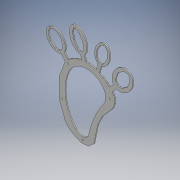
# Autodesk Inventor part: pata-carli
Saved by Autodesk Inventor 2018 (Build 220112000, 112)
## iProperties
Created: 2019-01-30
Part Number: pata-carli
Material: Generic
Document SubType Name: Modeling
Designer: Estudiante
Density: 1 g/cm^3
Appearance: Default
Author: Estudiante
Autodesk Inventor part; units mm, degrees
ref_plane "YZ Plane" through (0, 0, 0) normal (1, 0, 0) x (0, 1, 0)
ref_plane "XZ Plane" through (0, 0, 0) normal (0, 1, 0) x (-1, 0, 0)
ref_plane "XY Plane" through (0, 0, 0) normal (0, 0, 1) x (1, 0, 0)
sketch "Sketch1" plane through (0, 0, 0) normal (0, 1, 0) x (-1, 0, 0)
  line L0 (29.0554, 72.9814) -> (31.569, 71.953)
  line L1 (26.8219, 78.0587) -> (27.3884, 75.1254)
  line L2 (-19.8596, 89.1891) -> (-16.4882, 83.2487)
  line L3 (-14.1887, 81.7828) -> (-16.4882, 83.2487)
  line L4 (-11.9312, 81.6749) -> (-14.1887, 81.7828)
  line L5 (-10.0593, 82.9415) -> (-8.8581, 85.3896)
  line L6 (-11.9312, 81.6749) -> (-10.0593, 82.9415)
  line L7 (-8.8581, 85.3896) -> (-9.069, 92.2167)
  line L8 (-41.4432, 74.6738) -> (-35.9743, 70.6026)
  line L9 (-33.1014, 70.2673) -> (-35.9743, 70.6026)
  line L10 (-29.1988, 73.2448) -> (-28.7633, 76.1043)
  line L11 (-30.7221, 71.1952) -> (-33.1014, 70.2673)
  line L12 (-30.7221, 71.1952) -> (-29.1988, 73.2448)
  line L13 (-7.492, 12.8385) -> (-5.9259, 5.1471)
  line L14 (-9.7228, 24.2495) -> (-7.492, 12.8385)
  line L15 (-14.8718, 34.6743) -> (-9.7228, 24.2495)
  arc A0 (0, 8.9928) -> (-17.0107, 47.8982) centre (-95.643, -9.6539) ccw
  line L16 (-22.5775, 43.3812) -> (-14.8718, 34.6743)
  line L17 (31.569, 71.953) -> (34.5464, 72.1968)
  line L18 (29.1542, 84.4544) -> (26.8219, 78.0587)
  line L19 (34.5464, 72.1968) -> (40.0784, 76.1644)
  ellipse E0 centre (34.1936, 79.8506) end of major axis (26.5803, 71.3598) minor radius 9.1242 (28.5488, 70.094) -> (25.1982, 73.0271) ccw
  line L20 (40.0784, 76.1644) -> (42.4108, 82.5601)
  line L21 (34.6862, 88.422) -> (29.1542, 84.4544)
  line L22 (37.6637, 88.6658) -> (34.6862, 88.422)
  line L23 (42.4108, 82.5601) -> (41.8442, 85.4933)
  line L24 (38.9769, 87.7295) -> (37.6637, 88.6658)
  line L25 (41.8442, 85.4933) -> (40.5696, 86.5213)
  line L26 (9.0686, 82.2611) -> (11.3681, 83.5573)
  line L27 (4.8438, 86.2831) -> (5.5377, 83.7363)
  line L28 (12.3808, 100.1152) -> (10.0813, 98.819)
  line L29 (10.0813, 98.819) -> (6.1114, 93.1156)
  line L30 (13.4287, 100.083) -> (12.3808, 100.1152)
  line L31 (15.9117, 98.6399) -> (15.1525, 99.3628)
  line L32 (16.6056, 96.0931) -> (15.9117, 98.6399)
  line L33 (6.1114, 93.1156) -> (4.8438, 86.2831)
  ellipse E1 centre (10.6599, 91.6284) end of major axis (5.8794, 80.032) minor radius 8.4665 (8.3836, 79.5956) -> (4.3048, 81) ccw
  line L34 (15.3381, 89.2606) -> (16.6056, 96.0931)
  line L35 (11.3681, 83.5573) -> (15.3381, 89.2606)
  line L36 (6.6564, 75.1739) -> (11.5071, 73.874)
  line L37 (17.2873, 71.1447) -> (11.5071, 73.874)
  line L38 (21.4394, 68.1777) -> (17.2873, 71.1447)
  line L39 (21.4394, 68.1777) -> (17.2873, 71.1447)
  line L40 (25.1982, 73.0271) -> (21.4394, 68.1777)
  line L41 (29.0554, 72.9814) -> (27.3884, 75.1254)
  line L42 (28.5488, 70.094) -> (24.4313, 64.7818)
  line L43 (30.8467, 47.8624) -> (24.4313, 64.7818)
  line L44 (24.4313, 64.7818) -> (30.8467, 47.8624)
  line L45 (-43.9252, 81.0239) -> (-41.4432, 74.6738)
  line L46 (-28.7633, 76.1043) -> (-31.2452, 82.4543)
  ellipse E2 centre (-35.9971, 78.0469) end of major axis (-28.1232, 67.9201) minor radius 9.7067 (-26.561, 69.5776) -> (-29.6965, 66.9839) ccw
  line L47 (-43.4897, 83.8833) -> (-43.9252, 81.0239)
  line L48 (-31.2452, 82.4543) -> (-36.7141, 86.5255)
  line L49 (-42.5628, 85.1304) -> (-43.4897, 83.8833)
  line L50 (-36.7141, 86.5255) -> (-39.5871, 86.8608)
  line L51 (-39.5871, 86.8608) -> (-41.0347, 86.2963)
  ellipse E3 centre (-14.6571, 90.5791) end of major axis (-17.7823, 101.3962) minor radius 7.7041 (-10.1842, 80.3645) -> (-13.4664, 79.5698) ccw
  line L52 (-20.0705, 96.0162) -> (-19.8596, 89.1891)
  line L53 (-20.0705, 96.0162) -> (-19.8596, 89.1891)
  line L54 (-9.069, 92.2167) -> (-12.4404, 98.1571)
  line L55 (-12.4404, 98.1571) -> (-14.7399, 99.623)
  line L56 (-18.8693, 98.4643) -> (-20.0705, 96.0162)
  line L57 (-14.7399, 99.623) -> (-15.9985, 99.6831)
  line L58 (-17.8256, 99.1705) -> (-18.8693, 98.4643)
  line L59 (-26.561, 69.5776) -> (-22.2934, 65.085)
  line L60 (-19.5653, 67.6766) -> (-22.2934, 65.085)
  line L61 (-22.2934, 65.085) -> (-19.5653, 67.6766)
  line L62 (7.0212, 82.3239) -> (9.0686, 82.2611)
  line L63 (-1.0343, 75.4482) -> (2.443, 75.5931)
  arc A1 (20.9491, 56.7394) -> (-17.0336, 58.9292) centre (1.4249, 48.592) ccw
  line L64 (-1.0343, 75.4482) -> (-5.3277, 74.7251)
  line L65 (-5.3277, 74.7251) -> (-8.4472, 73.7874)
  line L66 (-10.1842, 80.3645) -> (-8.4472, 73.7874)
  line L67 (-11.7571, 72.5094) -> (-15.6173, 70.4963)
  line L68 (-13.4664, 79.5698) -> (-11.7571, 72.5094)
  line L69 (-15.6173, 70.4963) -> (-19.5653, 67.6766)
  line L70 (-5.9259, 5.1471) -> (0, 0)
  arc A2 (0, 8.9928) -> (13.4616, 9.0233) centre (6.7184, 14.472) ccw
  line L71 (0, 0) -> (7.8348, -0.474)
  line L72 (7.8348, -0.474) -> (13.896, 1.8858)
  arc A3 (13.4616, 9.0233) -> (20.9491, 56.7394) centre (-21.6227, 38.9742) ccw
  line L73 (30.8467, 28.3288) -> (30.8467, 47.8624)
  line L74 (23.9212, 10.0642) -> (30.8467, 28.3288)
  line L75 (19.3368, 5.4501) -> (23.9212, 10.0642)
  line L76 (13.896, 1.8858) -> (19.3368, 5.4501)
  line L77 (7.0212, 82.3239) -> (5.5377, 83.7363)
  line L78 (8.3836, 79.5956) -> (6.6564, 75.1739)
  line L79 (4.3048, 81) -> (2.443, 75.5931)
  line L80 (-29.6965, 66.9839) -> (-24.9466, 62.0994)
  line L81 (-24.9466, 62.0994) -> (-25.5349, 61.3378)
  line L82 (-25.5349, 61.3378) -> (-26.6253, 59.7519)
  line L83 (-26.6253, 59.7519) -> (-27.6265, 58.108)
  line L84 (-27.6265, 58.108) -> (-27.7405, 52.6995)
  line L85 (-27.7405, 52.6995) -> (-25.9861, 47.5821)
  line L86 (-25.9861, 47.5821) -> (-22.5775, 43.3812)
  circle A4 centre (-22.5775, 54.4696) radius 0.75
  arc A5 (-17.0336, 58.9292) -> (-17.0107, 47.8982) centre (-6.1714, 53.4362) ccw
  arc A6 (-41.0347, 86.2963) -> (-42.5628, 85.1304) centre (-41.9663, 85.933) ccw
  arc A7 (-15.9985, 99.6831) -> (-17.8256, 99.1705) centre (-16.9974, 99.7309) ccw
  arc A8 (15.1525, 99.3628) -> (13.4287, 100.083) centre (14.4282, 100.0523) ccw
  arc A9 (40.5696, 86.5213) -> (38.9769, 87.7295) centre (39.7912, 87.149) ccw
  circle A10 centre (5.6046, 2.8215) radius 0.75
  circle A11 centre (27.384, 29.6418) radius 0.75
  circle A12 centre (21.4394, 64.7818) radius 0.75
  point P0 (0, 0)
  point P1 (0, 0)
  point P2 (4.1459, 1.3104)
  dimension "d0" = 1.5
  dimension "d1" = 2
  dimension "d2" = 2
  dimension "d3" = 2
  dimension "d4" = 2
  dimension "d5" = 1.5
  dimension "d6" = 1.5
  dimension "d7" = 1.5
  constraints: 174 end point, 18 point on circle, 13 centre point, 1 parallel, 1 perpendicular, 1 tangent, 16 other
  measures "d0" diameter of A4
  measures "d1" diameter of A6
  measures "d2" diameter of A7
  measures "d3" diameter of A8
  measures "d4" diameter of A9
  measures "d5" diameter of A10
  measures "d6" diameter of A11
  measures "d7" diameter of A12
extrude "Extrusion1" add sketch "Sketch1" along normal blind 1
body "Solid1"
